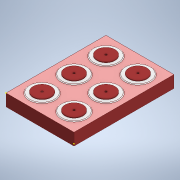
# Autodesk Inventor part: Część1
Saved by Autodesk Inventor 2020 (Build 240168000, 168)
## iProperties
Created: 2020-09-07
Part Number: Część1
Material: Ogólny
Document SubType Name: Modeling
Designer: szymon
Density: 1 g/cm^3
Appearance: Domyślna
Author: szymon
Autodesk Inventor part; units mm, degrees
ref_plane "YZ Plane" through (0, 0, 0) normal (1, 0, 0) x (0, 1, 0)
ref_plane "XZ Plane" through (0, 0, 0) normal (0, 1, 0) x (-1, 0, 0)
ref_plane "XY Plane" through (0, 0, 0) normal (0, 0, 1) x (1, 0, 0)
sketch "Szkic1" plane through (0, 0, 0) normal (0, 1, 0) x (-1, 0, 0)
  line L0 (0, 0) -> (-170, 0)
  line L1 (-170, 0) -> (-170, -250)
  line L2 (-170, -250) -> (0, -250)
  line L3 (0, -250) -> (0, 0)
  dimension "d0" = 170
  dimension "d1" = 250
  constraints: 8 end point, 2 parallel, 1 horizontal, 1 perpendicular
  measures "d0" distance of L2.end L1.end
  measures "d1" distance of L1.end L0.end
extrude "Wyciągnięcie proste1" add sketch "Szkic1" along normal blind 25
sketch "Szkic2" plane through (0, 25, 0) normal (0, 1, 0) x (1, 0, 0)
  circle A0 centre (45, 45) radius 22.5
  circle A1 centre (45, 45) radius 32.5
  circle A2 centre (45, 125) radius 32.5
  circle A3 centre (45, 125) radius 22.5
  circle A4 centre (45, 205) radius 32.5
  circle A5 centre (45, 205) radius 22.5
  circle A6 centre (45, 45) radius 2.5
  circle A7 centre (45, 125) radius 2.5
  circle A8 centre (45, 205) radius 2.5
  circle A9 centre (125, 45) radius 32.5
  circle A10 centre (125, 45) radius 22.5
  circle A11 centre (125, 125) radius 22.5
  circle A12 centre (125, 125) radius 32.5
  circle A13 centre (125, 205) radius 22.5
  circle A14 centre (125, 205) radius 32.5
  circle A15 centre (125, 45) radius 2.5
  circle A16 centre (125, 125) radius 2.5
  circle A17 centre (125, 205) radius 2.5
  point P0 (0, 0)
  dimension "d4" = 45
  dimension "d5" = 65
  dimension "d6" = 65
  dimension "d7" = 45
  dimension "d8" = 65
  dimension "d9" = 45
  dimension "d10" = 5
  dimension "d11" = 5
  dimension "d12" = 5
  dimension "d13" = 65
  dimension "d14" = 45
  dimension "d15" = 45
  dimension "d16" = 65
  dimension "d17" = 45
  dimension "d18" = 65
  dimension "d19" = 5
  dimension "d20" = 5
  dimension "d21" = 5
  constraints: 18 centre point, 12 coincident
  measures "d4" diameter of A0
  measures "d5" diameter of A1
  measures "d6" diameter of A2
  measures "d7" diameter of A3
  measures "d8" diameter of A4
  measures "d9" diameter of A5
  measures "d10" diameter of A6
  measures "d11" diameter of A7
  measures "d12" diameter of A8
  measures "d13" diameter of A9
  measures "d14" diameter of A10
  measures "d15" diameter of A11
  measures "d16" diameter of A12
  measures "d17" diameter of A13
  measures "d18" diameter of A14
  measures "d19" diameter of A15
  measures "d20" diameter of A16
  measures "d21" diameter of A17
extrude "Wyciągnięcie proste2" add sketch "Szkic2" along normal blind 3 contours A0 | A3 | A5 | A10 | A11 | A13
sketch "Szkic3" plane through (45, 25, -45) normal (0, 1, 0) x (1, 0, 0)
  circle A0 centre (0, 0) radius 32.5
  circle A1 centre (0, 80) radius 2.5 projected
  circle A2 centre (0, 80) radius 32.5
  circle A3 centre (0, 160) radius 2.5 projected
  circle A4 centre (0, 160) radius 32.5
  circle A5 centre (80, 0) radius 2.5 projected
  circle A6 centre (80, 0) radius 32.5
  circle A7 centre (80, 80) radius 2.5 projected
  circle A8 centre (80, 80) radius 32.5
  circle A9 centre (80, 160) radius 2.5 projected
  circle A10 centre (80, 160) radius 32.5
  point P0 (-45, -45)
  dimension "d24" = 65
  dimension "d25" = 65
  dimension "d26" = 65
  dimension "d27" = 65
  dimension "d28" = 65
  dimension "d29" = 65
  constraints: 6 centre point, 5 coincident
  measures "d24" diameter of A0
  measures "d25" diameter of A2
  measures "d26" diameter of A4
  measures "d27" diameter of A6
  measures "d28" diameter of A8
  measures "d29" diameter of A10
extrude "Wyciągnięcie proste3" add sketch "Szkic3" along normal blind 1.5
fillet "Zaokrąglenie1" radius 2 1 edges at (12.5, 26.5, -45)
fillet "Zaokrąglenie2" radius 2 1 edges at (12.5, 26.5, -125)
fillet "Zaokrąglenie3" radius 2 1 edges at (12.5, 26.5, -205)
fillet "Zaokrąglenie4" radius 2 3 edges at (92.5, 26.5, -205) (92.5, 26.5, -125) (92.5, 26.5, -45)
sketch "Szkic4" plane through (125, 25, -45) normal (0, 1, 0) x (1, 0, 0)
  circle A0 centre (-80.0767, -0.0437) radius 2.585
  circle A1 centre (-80.0767, 79.8638) radius 0.5362
  point P0 (-125, -45)
  constraints: 2 centre point
sketch "Szkic5" plane through (0, 0, 0) normal (0, -1, 0) x (1, 0, 0)
  line L0 (0, 0) -> (170, 0) projected
  line L1 (170, -250) -> (0, -250) projected
  line L2 (170, 0) -> (0, 0)
  line L3 (0, 0) -> (0, -250)
  line L4 (0, -250) -> (170, -250)
  line L5 (170, -250) -> (170, 0)
  constraints: 8 end point, 2 parallel, 1 horizontal, 1 perpendicular
extrude "Wyciągnięcie proste4" add sketch "Szkic5" along normal blind 5
sketch "Szkic6" plane through (170, 25, 0) normal (1, 0, 0) x (0, 0, -1)
  point P0 (0, -25)
